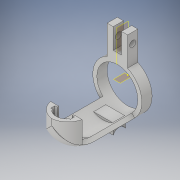
# Autodesk Inventor part: beta_dummy
Saved by Autodesk Inventor 2018 (Build 220112000, 112)
## iProperties
Created: 2017-10-07
Part Number: beta_dummy
Material: Generic
Document SubType Name: Modeling
Designer: rheal
Density: 1 g/cm^3
Appearance: Default
Author: rheal
Autodesk Inventor part; units mm, degrees
ref_plane "YZ Plane" through (0, 0, 0) normal (1, 0, 0) x (0, 1, 0)
ref_plane "XZ Plane" through (0, 0, 0) normal (0, 1, 0) x (-1, 0, 0)
ref_plane "XY Plane" through (0, 0, 0) normal (0, 0, 1) x (1, 0, 0)
sketch "Sketch1" plane through (0, 0, 0) normal (0, 0, 1) x (1, 0, 0)
  arc A0 (6.000593, 0.076915) -> (5.99995, -0.024489) centre (14, -0.024489) ccw
  line L0 (-5, 20) -> (-5, 5.908712)
  line L1 (0, 10) -> (0, 17.055195) construction
  line L2 (5, 20) -> (5, 5.908712)
  circle A1 centre (0, -5) radius 10
  arc A2 (-5, 5.908712) -> (5, 5.908712) centre (0, -5) ccw
  line L3 (5, 10) -> (-5, 10) construction
  line L4 (0, 10) -> (0, 20) construction
  line L5 (-1.5, 20) -> (-1.5, 10)
  line L6 (1.5, 20) -> (1.5, 10)
  line L7 (5, 20) -> (1.5, 20)
  line L8 (-1.5, 20) -> (-5, 20)
  line L9 (-1.5, 10) -> (1.5, 10)
  point P0 (0, 0)
  point P1 (8, 0)
  dimension "d24" = 20
  dimension "d46" = 1.5
  constraints: 20 end point, 4 point on circle, 3 centre point, 3 perpendicular, 3 point on line, 3 symmetric about line, 3 vertical, 1 coincident, 1 collinear, 1 horizontal
  measures "d24" diameter of A1
  measures "d46" distance of L4.end L5.start
extrude "Extrusion1" add sketch "Sketch1" along normal blind 5
sketch "Sketch3" plane through (0, 0, 5) normal (0, 0, 1) x (1, 0, 0)
  circle A0 centre (0, -5) radius 10
  point P0 (0, 0)
  dimension "d26" = 20
  constraints: 1 centre point
  measures "d26" diameter of A0
extrude "Extrusion3" cut sketch "Sketch3" against normal blind 5
sketch "Sketch4" plane through (5, 5.908712, 0) normal (1, 0, 0) x (0, 0, -1)
  line L0 (0, 14.091288) -> (-5, 14.091288) construction
  line L1 (-2.5, 14.091288) -> (-2.5, 9.091288) construction
  circle A0 centre (-2.5, 9.091288) radius 1.5
  point P0 (0, -5.908712)
  dimension "d30" = 5
  dimension "d31" = 3
  constraints: 2 end point, 1 centre point, 1 coincident, 1 midpoint, 1 vertical
  measures "d30" distance of L1.start L1.end
  measures "d31" diameter of A0
extrude "Extrusion4" cut sketch "Sketch4" against normal blind 10
ref_plane "Work Plane1" through (0, 5.908712, 0) normal (1, 0, 0) x (0, 0, -1)
sketch "Sketch7" plane through (0, 5.908712, 0) normal (1, 0, 0) x (0, 0, -1)
  line L0 (-5, -20.908712) -> (-5, -0.908712) construction
  line L1 (-5, -20.908712) -> (-25, -20.908712)
  line L2 (-5, -0.908712) -> (-5, -20.908712) construction
  line L3 (0, 0) -> (0, -22.908712)
  line L4 (-5, -10.908712) -> (-25, -10.908712) construction
  line L5 (-5, -22.908712) -> (-25, -22.908712)
  line L6 (-5, 0) -> (-5, -22.908712)
  line L7 (-5, -20.908712) -> (-5, -22.908712)
  arc A0 (-37, -10.908712) -> (-25, -22.908712) centre (-25, -10.908712) ccw
  arc A1 (-35, -10.908712) -> (-25, -20.908712) centre (-25, -10.908712) ccw
  line L8 (-35, -10.908712) -> (-37, -10.908712)
  point P0 (0, -5.908712)
  constraints: 12 end point, 4 point on circle, 3 horizontal, 2 centre point, 2 coincident, 2 parallel, 1 midpoint, 1 vertical
revolve "Revolution1" add sketch "Sketch7" angle 90 mid plane about axis through (0, -5, 5) along (0, 0, 1)
ref_plane "Work Plane2" through (-1.5, -2, 0) normal (0, 1, 0) x (1, 0, 0)
sketch "Sketch8" plane through (-1.5, -2, 0) normal (0, 1, 0) x (1, 0, 0)
  ellipse E0 centre (1.5, -25) end of major axis (1.5, -15) minor radius 7.071068 (1.5, -35) -> (8.571068, -25) ccw
  line L0 (1.5, -25) -> (1.5, -30)
  line L1 (1.5, -30) -> (11.626354, -30)
  line L2 (1.5, -30) -> (1.5, -35)
  arc A0 (1.5, -35) -> (7.623724, -30) centre (0.83072, -27.930303) ccw
  line L3 (1.5, -35) -> (1.5, -37)
  line L4 (1.5, -35) -> (1.5, -37)
  ellipse E1 centre (1.5, -25) end of major axis (1.5, -37) minor radius 8.485281 (1.5, -37) -> (9.985281, -25) ccw
  arc A1 (1.5, -37) -> (9.213624, -30) centre (0.49458, -28.142081) ccw
  line L5 (7.623724, -30) -> (5.123724, -30)
  line L6 (5.123724, -30) -> (5.123724, -33.587039)
  line L7 (5.123724, -33.587039) -> (7.623724, -33.587039)
  line L8 (7.623724, -33.587039) -> (7.623724, -30)
  point P0 (1.5, 0)
  dimension "d49" = 5
  dimension "d68" = 2.5
  constraints: 16 end point, 5 point on circle, 3 vertical, 2 centre point, 2 parallel, 2 perpendicular, 2 point on line, 1 horizontal, 5 other
  measures "d49" distance of L0.start L0.end
  measures "d68" distance of L6.end L7.end
sketch "Sketch8 outline for Extrusion6" plane through (-1.5, -2, 0) normal (0, 1, 0) x (1, 0, 0)
  spline S0 degree 2 poles (1.5, -35) (3.449597, -35) (5.123724, -33.587039) knots 0 0 0 1 1 1 weights 1 0.96402903 1
  line L0 (1.5, -35) -> (1.5, -37)
  arc A0 (1.5, -37) -> (9.213624, -30) centre (0.49458, -28.142081) ccw
  line L1 (9.213624, -30) -> (5.123724, -30)
  line L2 (5.123724, -30) -> (5.123724, -33.587039)
extrude "Extrusion6" add sketch "Sketch8 outline for Extrusion6" against normal up to surface surface through (6.523113, -11.523113, 21.638928) normal (0.7071068, 0.7071068, 0)
sketch "Sketch9" plane through (-1.5, -2, 0) normal (0, 1, 0) x (1, 0, 0)
  point P0 (1.5, 0)
sketch "Sketch10" plane through (-1.5, -2, 0) normal (0, 1, 0) x (1, 0, 0)
  line L0 (3.998724, -32.79352) -> (6.248724, -32.79352)
  line L1 (6.248724, -32.79352) -> (6.248724, -30.79352)
  line L2 (6.248724, -30.79352) -> (3.998724, -30.79352)
  line L3 (3.998724, -30.79352) -> (3.998724, -32.79352)
  line L4 (5.123724, -30) -> (5.123724, -33.587039)
  line L5 (3.998724, -32.79352) -> (6.248724, -30.79352) construction
  line L6 (6.248724, -32.79352) -> (3.998724, -30.79352) construction
  point P0 (1.5, 0)
  point P1 (5.123724, -31.79352)
  dimension "d52" = 2.25
  dimension "d53" = 2
  constraints: 12 end point, 3 midpoint, 2 parallel, 1 horizontal, 1 perpendicular
  measures "d52" distance of L2.end L1.end
  measures "d53" distance of L1.end L0.end
extrude "Extrusion7" cut sketch "Sketch10" against normal blind 5
sketch "Sketch11" plane through (4.748724, -2, 30.79352) normal (-1, 0, 0) x (0, 0, 1)
  line L0 (2, -5) -> (0, -5) projected
  line L1 (1, -5) -> (1, -3)
  circle A0 centre (1, -4) radius 1
  point P0 (-30.79352, 2)
  dimension "d56" = 2
  constraints: 2 end point, 2 midpoint, 1 centre point, 1 vertical
  measures "d56" distance of L1.start L1.end
sketch "Sketch11 outline for Extrusion8" plane through (4.748724, -2, 30.79352) normal (-1, 0, 0) x (0, 0, 1)
  circle A0 centre (1, -4) radius 1
extrude "Extrusion8" cut sketch "Sketch11 outline for Extrusion8" against normal blind 0.75 draft -30
mirror "Mirror1" about plane through (0, -2, 37) normal (-1, 0, 0) of "Extrusion6", "Extrusion8", "Extrusion7"
sketch "Sketch12" plane through (5, 5.908712, 0) normal (1, 0, 0) x (0, 0, -1)
  line L0 (0, -22.908712) -> (-6, -22.908712)
  line L1 (-12, -22.908712) -> (-12, -24.908712)
  line L2 (-6, -22.908712) -> (-6, -24.908712)
  arc A0 (-6, -24.908712) -> (-12, -24.908712) centre (-9, -26.158712) ccw
  line L3 (-12, -22.908712) -> (-12, -19.768037)
  line L4 (-12, -19.768037) -> (-6, -19.768037)
  line L5 (-6, -19.768037) -> (-6, -22.908712)
  point P0 (0, -5.908712)
  dimension "d59" = 6
  dimension "d61" = 2
  constraints: 12 end point, 2 perpendicular, 2 point on circle, 1 centre point, 1 vertical
  measures "d59" distance of L0.start L0.end
  measures "d61" distance of L1.start L1.end
extrude "Extrusion9" add sketch "Sketch12" against normal blind 10
sketch "Sketch13" plane through (0, 0, 5) normal (0, 0, 1) x (1, 0, 0)
  line L0 (-2, 20) -> (2, 20)
  line L1 (2, 20) -> (2, 10)
  line L2 (2, 10) -> (-2, 10)
  line L3 (-2, 10) -> (-2, 20)
  line L4 (-2, 20) -> (2, 10) construction
  line L5 (2, 20) -> (-2, 10) construction
  point P0 (0, 0)
  point P1 (0, 15)
  dimension "d65" = 4
  constraints: 12 end point, 2 midpoint, 2 parallel, 1 horizontal, 1 perpendicular
  measures "d65" distance of L1.end L2.end
extrude "Extrusion10" cut sketch "Sketch13" against normal through all
body "Solid1"
